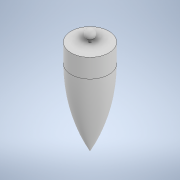
# Autodesk Inventor part: octopus tentacle end
Saved by Autodesk Inventor 2021 (Build 250183000, 183)
## iProperties
Created: 2020-07-11
Part Number: octopus tentacle end
Material: Generic
Document SubType Name: Modeling
Designer: saipr
Density: 1 g/cm^3
Appearance: Default
Mass: 20.589 g
Surface Area: 44.4948 cm^2
Volume: 20.589 cm^3
Author: saipr
Autodesk Inventor part; units mm, degrees
ref_plane "YZ Plane" through (0, 0, 0) normal (1, 0, 0) x (0, 1, 0)
ref_plane "XZ Plane" through (0, 0, 0) normal (0, 1, 0) x (-1, 0, 0)
ref_plane "XY Plane" through (0, 0, 0) normal (0, 0, 1) x (1, 0, 0)
sketch "Sketch1" plane through (0, 0, 0) normal (0, 0, 1) x (1, 0, 0)
  circle A0 centre (0, 0) radius 3.175
  line L0 (0, 0) -> (3.175, 0)
  line L1 (0, 0) -> (0, -3.175)
  line L2 (0, 0) -> (2.2451, -2.2451)
  line L3 (0, 0) -> (-2.2451, -2.2451)
  line L4 (0, 0) -> (-3.175, 0)
  line L5 (-1.5875, 0) -> (0, 0)
  line L6 (0, 0) -> (1.5875, 0)
  line L7 (0, 0) -> (-0.7938, 0)
  line L8 (0, 0) -> (0.7937, 0)
  line L9 (-0.7938, 0) -> (-0.7938, -7.5506)
  line L10 (-0.7938, -7.5506) -> (0.7937, -7.5506)
  line L11 (0.7937, -7.5506) -> (0.7937, 0)
  arc A1 (-0.7938, -5.1785) -> (-2.2451, -2.2451) centre (-4.4839, -5.1785) ccw
  arc A2 (2.2451, -2.2451) -> (0.7937, -5.1785) centre (4.4839, -5.1785) ccw
  line L12 (0, 3.175) -> (0, -7.5506)
  line L13 (-0.7938, -5.1785) -> (0.7937, -5.1785)
  line L14 (-0.7938, -5.1785) -> (-3.1545, -5.1785)
  line L15 (0.7937, -5.1785) -> (3.1408, -5.1785)
  line L16 (-0.0063, -5.1785) -> (13.6859, -5.1785)
  line L17 (13.6859, -5.1785) -> (13.6859, -18.8349)
  line L18 (13.6859, -18.8349) -> (-0.0064, -18.8349)
  line L19 (-0.0063, -5.1785) -> (-13.6859, -5.1785)
  line L20 (-13.6859, -5.1785) -> (-13.6859, -18.8349)
  line L21 (-13.6859, -18.8349) -> (-0.0064, -18.8349)
  arc A3 (-13.6859, -18.8349) -> (0, -73.864) centre (103.7891, -18.8349) ccw
  arc A4 (0, -73.864) -> (13.6859, -18.8349) centre (-103.7891, -18.8349) ccw
  line L22 (0, -7.5506) -> (0, -73.864)
  line L23 (-13.6859, -18.8349) -> (-10.5109, -18.8349)
  line L24 (13.6859, -18.8349) -> (10.5109, -18.8349)
  line L25 (-13.6859, -5.1785) -> (-13.6859, -8.3535)
  line L26 (-10.5109, -18.8349) -> (-10.5109, -8.3535)
  line L27 (-10.5109, -8.3535) -> (10.5109, -8.3535)
  line L28 (10.5109, -8.3535) -> (10.5109, -18.8349)
  line L29 (0, -73.864) -> (0, -70.689)
  arc A5 (-10.5109, -18.8349) -> (0, -70.689) centre (106.9208, -22.0236) ccw
  arc A6 (0, -70.689) -> (10.5109, -18.8349) centre (-106.9208, -22.0236) ccw
  point P0 (0, 0)
  point P1 (0, -3.175)
  point P2 (1.5373, -5.4355)
  point P3 (0, -5.1785)
  point P4 (0.7937, 0)
  point P5 (0, -8.3535)
  dimension "d0" = 6.35
  dimension "d1" = 45
  dimension "d2" = 45
  dimension "d3" = 7.5506
  dimension "d17" = 13.6564
  dimension "d18" = 5.1785
  dimension "d20" = 13.6922
  dimension "d21" = 13.6796
  dimension "d22" = 117.475
  dimension "d23" = 117.475
  dimension "d27" = 3.175
  dimension "d28" = 3.175
  dimension "d29" = 3.175
  dimension "d30" = 10.4814
  dimension "d31" = 3.175
  dimension "d32" = 117.475
  dimension "d33" = 117.475
  constraints: 60 end point, 18 point on circle, 9 perpendicular, 8 point on line, 7 centre point, 5 horizontal, 5 midpoint, 4 tangent, 3 vertical, 2 parallel, 1 coincident
  measures "d0" diameter of A0
  measures "d1" angle of L0 L2
  measures "d2" angle of L3 L4
  measures "d3" distance of L10.end L8.end
  measures "d17" distance of L16.end L17.end
  measures "d18" distance from line of L16 L0.start
  measures "d20" distance of L16.start L16.end
  measures "d21" distance of L16.start L19.end
  measures "d22" radius of A4
  measures "d23" radius of A3
  measures "d27" distance of L20.end L23.end
  measures "d28" distance of L17.end L24.end
  measures "d29" distance of L19.end L25.end
  measures "d30" distance of L27.end L24.end
  measures "d31" distance of L22.end L29.end
  measures "d32" radius of A5
  measures "d33" radius of A6
revolve "Revolution2" add sketch "Sketch1" angle 360 about axis through (0, 3.175, 0) along (0, -1, 0) contours L0 L12 A0 | A0 L2 L11 L0 | A2 A0 L11 L2 | L2 L11 A0 L1 | L0 L11 L2 | A2 L11 A0 | A0 L11 L13 L12 | L15 L16 L17 L18 L28 L27 L22 L10 L11 | L11 L10 L12 L13 | A4 L22 A6 L18
equation "\"d32\" = d23"
equation "\"d33\" = d23"
body "Solid2"
